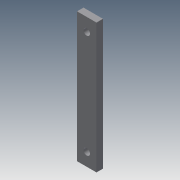
# Autodesk Inventor part: mallet_sideplate
Saved by Autodesk Inventor 2015 (Build 190159000, 159)
## iProperties
Created: 2014-08-31
Part Number: mallet_sideplate
Material: Generic
Document SubType Name: Modeling
Designer: shohei
Density: 1 g/cm^3
Appearance: Default
Author: shohei
Autodesk Inventor part; units mm, degrees
ref_plane "YZ Plane" through (0, 0, 0) normal (1, 0, 0) x (0, 1, 0)
ref_plane "XZ Plane" through (0, 0, 0) normal (0, 1, 0) x (-1, 0, 0)
ref_plane "XY Plane" through (0, 0, 0) normal (0, 0, 1) x (1, 0, 0)
sketch "Sketch1" plane through (0, 0, 0) normal (0, 1, 0) x (-1, 0, 0)
  line L0 (0, 0) -> (30, 0)
  line L1 (30, 0) -> (30, 200)
  line L2 (30, 200) -> (0, 200)
  line L3 (0, 200) -> (0, 0)
  circle A0 centre (15, 180) radius 5
  circle A1 centre (15, 20) radius 5
  dimension "d0" = 30
  dimension "d1" = 200
  dimension "d2" = 10
  dimension "d3" = 10
  dimension "d4" = 20
  dimension "d5" = 20
  constraints: 8 end point, 2 centre point, 2 parallel, 1 horizontal, 1 perpendicular
  measures "d0" distance of L1.end L2.end
  measures "d1" distance of L0.end L1.end
  measures "d2" diameter of A0
  measures "d3" diameter of A1
  measures "d4" distance from line of L0 A1.centre
  measures "d5" distance from line of L2 A0.centre
extrude "Extrusion1" add sketch "Sketch1" along normal blind 10
body "Solid1"
